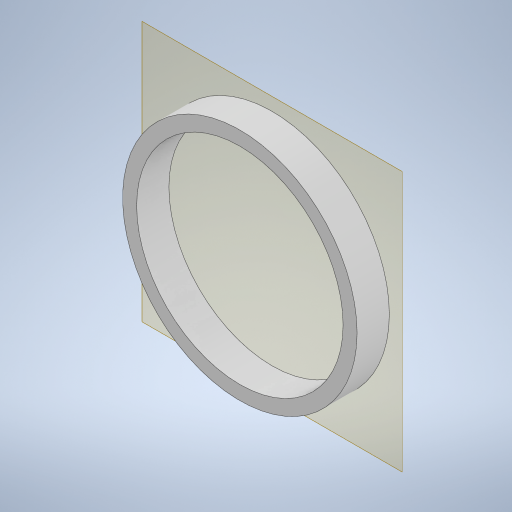
# Autodesk Inventor part: bearing-spacer-top
Saved by Autodesk Inventor 2024 (Build 280153000, 153)
## iProperties
Created: 2024-04-10
Part Number: bearing-spacer-top
Material: Generic
Document SubType Name: Modeling
Designer: MaartenGeorgesBuelen
Density: 1 g/cm^3
Appearance: Default
Author: MaartenGeorgesBuelen
## iProperties of the stored document bearing-spacer-top_3DPrint.ipt
Created: 2024-04-10
Part Number: bearing-spacer-top_3DPrint
Material: Generic
Document SubType Name: Modeling
Designer: MaartenGeorgesBuelen
Density: 1 g/cm^3
Appearance: Default
Author: MaartenGeorgesBuelen
Autodesk Inventor part; units mm, degrees
ref_plane "YZ Plane" through (0, 0, 0) normal (1, 0, 0) x (0, 1, 0)
ref_plane "XZ Plane" through (0, 0, 0) normal (0, 1, 0) x (-1, 0, 0)
ref_plane "XY Plane" through (0, 0, 0) normal (0, 0, 1) x (1, 0, 0)
ref_plane "Work Plane1" through (0, 0, 0) normal (0, 0, 1) x (1, 0, 0)
sketch "Sketch1" plane through (0, 0, 0) normal (0, 0, 1) x (1, 0, 0)
  circle A0 centre (0, 0) radius 19
  arc A1 (20.75769, 7.28823) -> (-20.75769, 7.28823) centre (0, 0) ccw
  circle A2 centre (0, 0) radius 15
  circle A3 centre (0, 0) radius 22
  circle A4 centre (0, 0) radius 21.8
  circle A5 centre (0, 0) radius 19.2
  point P0 (0, 0)
  dimension "d0" = 0.2
  dimension "d1" = 0.2
  constraints: 2 centre point
  measures "d0" radial gap between concentric circles of A3 A4
  measures "d1" radial gap between concentric circles of A0 A5
sketch "Sketch1 outline for Extrusion1" plane through (0, 0, 0) normal (0, 0, 1) x (1, 0, 0)
  circle A0 centre (0, 0) radius 21.8
  circle A1 centre (0, 0) radius 19.2
extrude "Extrusion1" add sketch "Sketch1 outline for Extrusion1" along normal blind 6
body "Solid1"
